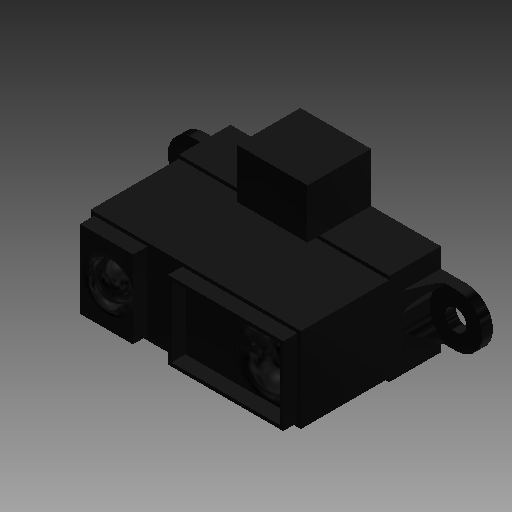
# Autodesk Inventor part: PSD
Saved by Autodesk Inventor 2017 (Build 210142000, 142)
## iProperties
Created: 2011-08-11
Part Number: PSD
Document SubType Name: Modeling
Designer: user
Density: 1.0545 g/cm^3
Mass: 5 g
Surface Area: 26.4147 cm^2
Volume: 4.74158 cm^3
Material: 알루미늄-6061
Appearance: 광택 - 검은색
Author: user
Autodesk Inventor part; units mm, degrees
ref_plane "YZ Plane" through (0, 0, 0) normal (1, 0, 0) x (0, 1, 0)
ref_plane "XZ Plane" through (0, 0, 0) normal (0, 1, 0) x (-1, 0, 0)
ref_plane "XY Plane" through (0, 0, 0) normal (0, 0, 1) x (1, 0, 0)
sketch "스케치1" plane through (0, 0, 0) normal (0, 0, 1) x (1, 0, 0)
  line L0 (0, 0) -> (-29.75, 0)
  line L1 (-29.75, 13) -> (0, 13)
  arc A0 (3.625, 2.75) -> (3.625, 10.25) centre (3.625, 6.5) ccw
  circle A1 centre (-33.375, 6.5) radius 1.5
  circle A2 centre (3.625, 6.5) radius 1.5
  line L2 (-0.25, 6.5) -> (0, 6.5)
  line L3 (-0.25, 6.5) -> (0, 6.5)
  line L4 (-37.125, 6.5) -> (-34.875, 6.5)
  line L5 (-29.5, 6.5) -> (-29.25, 6.5)
  line L6 (-29.75, 0) -> (-29.75, 2.75)
  line L7 (-29.75, 10.25) -> (-29.75, 13)
  arc A3 (-33.375, 10.25) -> (-33.375, 2.75) centre (-33.375, 6.5) ccw
  line L8 (-33.375, 10.25) -> (-29.75, 10.25)
  line L9 (0, 10.25) -> (3.625, 10.25)
  line L10 (3.625, 2.75) -> (0, 2.75)
  line L11 (-29.75, 2.75) -> (-33.375, 2.75)
  line L12 (0, 13) -> (0, 10.25)
  line L13 (0, 2.75) -> (0, 0)
  line L14 (5.125, 6.5) -> (7.375, 6.5)
  point P0 (-14.75, 6.5)
  point P1 (-14.75, 6.5)
  dimension "d5" = 3
  dimension "d56" = 3
  dimension "d0" = 29.75
  dimension "d1" = 13
  dimension "d3" = 7.5
  dimension "d4" = 44.5
  dimension "d53" = 29.75
  dimension "d54" = 2.125
  dimension "d55" = 2.125
  constraints: 30 end point, 9 parallel, 6 perpendicular, 6 point on circle, 3 horizontal, 2 centre point, 2 coincident, 2 horizontal alignment, 4 other
  measures "d0" distance of L1.start L1.end
  measures "d1" distance of L1.end L0.start
  measures "d3" diameter of A0
  measures "d4" distance of L4.start L14.end
  measures "d53" distance between parallel lines of L13 L6
extrude "돌출1" add sketch "스케치1" along normal blind 7.3
sketch "스케치2" plane through (0, 0, 7.3) normal (0, 0, 1) x (1, 0, 0)
  circle A0 centre (3.625, 6.5) radius 1.5 projected
  circle A1 centre (-33.375, 6.5) radius 1.5 projected
  line L0 (-29.75, 10.25) -> (-37, 10.25)
  line L1 (-37, 10.25) -> (-37, 0.8683)
  line L2 (-37, 0.8683) -> (-29.75, 0.8683)
  line L3 (-29.75, 0.8683) -> (-29.75, 10.25)
  line L4 (0, 10.25) -> (7.9641, 10.25)
  line L5 (7.9641, 10.25) -> (7.9641, 2.75)
  line L6 (7.9641, 2.75) -> (0, 2.75)
  line L7 (0, 2.75) -> (0, 10.25)
  constraints: 16 end point, 4 parallel, 2 horizontal, 2 perpendicular
extrude "돌출2" cut sketch "스케치2" against normal blind 5.8
chamfer "모따기1" distance 2 angle 45 2 edges at (0, 6.5, 1.5) (-29.75, 6.5, 1.5)
chamfer "모따기2" distance 2 angle 45 2 edges at (-29.75, 6.5, 3.5) (0, 6.5, 3.5)
sketch "스케치3" plane through (0, 0, 7.3) normal (0, 0, 1) x (1, 0, 0)
  line L0 (0, 13) -> (0, 0) projected
  line L1 (-29.75, 0) -> (-29.75, 13) projected
  line L2 (-29.75, 6.5) -> (0, 6.5)
  line L3 (0, 6.5) -> (0, 12.5)
  line L4 (0, 12.5) -> (-29.75, 12.5)
  line L5 (-29.75, 12.5) -> (-29.75, 6.5)
  line L6 (0, 12.5) -> (-29.75, 12.5)
  line L7 (-29.75, 12.5) -> (-29.75, 0.5)
  line L8 (-29.75, 0.5) -> (0, 0.5)
  line L9 (0, 0.5) -> (0, 12.5)
  dimension "d17" = 6
  dimension "d57" = 6
  constraints: 16 end point, 4 parallel, 2 horizontal, 2 perpendicular, 2 point on line, 1 midpoint
  measures "d17" distance of L4.end L2.start
  measures "d57" distance between parallel lines of L8 L2
extrude "돌출3" add sketch "스케치3" along normal blind 14.5
sketch "스케치4" plane through (0, 0, 21.8) normal (0, 0, 1) x (1, 0, 0)
  line L0 (-29.75, 0.5) -> (-29.75, 12.5) projected
  line L1 (0, 0.5) -> (-29.75, 0.5) projected
  line L2 (0, 12.5) -> (0, 0.5) projected
  line L3 (-29.75, 12.5) -> (0, 12.5) projected
  line L4 (-29.25, 12) -> (-0.5, 12)
  line L5 (-0.5, 12) -> (-0.5, 1)
  line L6 (-0.5, 1) -> (-29.25, 1)
  line L7 (-29.25, 1) -> (-29.25, 12)
  line L8 (-29.25, 12) -> (-21.75, 12)
  line L9 (-21.75, 12) -> (-21.75, 1)
  line L10 (-21.75, 1) -> (-29.25, 1)
  line L11 (-29.25, 1) -> (-29.25, 12)
  line L12 (-0.5, 12) -> (-16.8, 12)
  line L13 (-16.8, 12) -> (-16.8, 1)
  line L14 (-16.8, 1) -> (-0.5, 1)
  line L15 (-0.5, 1) -> (-0.5, 12)
  point P0 (0, 0)
  dimension "d22" = 0.5
  dimension "d23" = 0.5
  dimension "d24" = 0.5
  dimension "d25" = 0.5
  dimension "d26" = 7.5
  dimension "d27" = 16.3
  constraints: 24 end point, 6 parallel, 3 horizontal, 3 perpendicular, 2 point on line
  measures "d22" distance between parallel lines of L2 L5
  measures "d23" distance between parallel lines of L0 L7
  measures "d24" distance between parallel lines of L6 L1
  measures "d25" distance between parallel lines of L3 L4
  measures "d26" distance of L4.start L8.end
  measures "d27" distance of L4.end L12.end
extrude "돌출4" cut sketch "스케치4" against normal blind 2 contours L0 L3 L2 L1 | L4 L13 L6 L9
sketch "스케치5" plane through (0, 0, 21.8) normal (0, 0, 1) x (1, 0, 0)
  line L0 (-0.5, 1) -> (-0.5, 12) projected
  line L1 (-0.5, 12) -> (-16.8, 12) projected
  line L2 (-16.8, 12) -> (-16.8, 1) projected
  line L3 (-16.8, 1) -> (-0.5, 1) projected
  line L4 (-16.3, 11.5) -> (-1, 11.5)
  line L5 (-1, 11.5) -> (-1, 1.5)
  line L6 (-1, 1.5) -> (-16.3, 1.5)
  line L7 (-16.3, 1.5) -> (-16.3, 11.5)
  line L8 (-29.25, 1) -> (-21.75, 1) projected
  line L9 (-21.75, 1) -> (-21.75, 12) projected
  line L10 (-21.75, 12) -> (-29.25, 12) projected
  line L11 (-29.25, 12) -> (-29.25, 1) projected
  circle A0 centre (-25.25, 6.5) radius 2.75
  point P0 (0, 0)
  dimension "d30" = 0.5
  dimension "d31" = 0.5
  dimension "d32" = 0.5
  dimension "d33" = 0.5
  dimension "d34" = 5.5
  constraints: 8 end point, 2 parallel, 1 centre point, 1 horizontal, 1 perpendicular
  measures "d30" distance between parallel lines of L0 L5
  measures "d31" distance between parallel lines of L1 L4
  measures "d32" distance between parallel lines of L7 L2
  measures "d33" distance between parallel lines of L6 L3
  measures "d34" diameter of A0
extrude "돌출5" cut sketch "스케치5" against normal blind 2 contours L4 L5 L6 L7 | A0
fillet "모깎기1" radius 1 1 edges at (-28, 6.5, 21.8)
sketch "스케치6" plane through (0, 0, 19.8) normal (0, 0, 1) x (1, 0, 0)
  line L0 (-1, 1.5) -> (-1, 11.5) projected
  circle A0 centre (-4.2, 6.5) radius 2.75
  point P0 (0, 0)
  dimension "d38" = 5.5
  dimension "d39" = 3.2
  constraints: 1 centre point
  measures "d38" diameter of A0
  measures "d39" distance from line of L0 A0.centre
extrude "돌출6" cut sketch "스케치6" against normal blind 4
fillet "모깎기2" radius 3 1 edges at (-6.95, 6.5, 19.8)
sketch "스케치7" plane through (-4.2, 6.5, 15.8) normal (0, 0, 1) x (1, 0, 0)
  circle A0 centre (0, 0) radius 2.75 projected
  line L0 (-2.75, 0) -> (2.75, 0)
  point P0 (4.2, -6.5)
  constraints: 2 end point, 2 point on circle, 1 horizontal
revolve "회전1" add sketch "스케치7" angle 360 about axis through (-6.95, 6.5, 15.8) along (1, 0, 0) picked at (-1.0422, 1.0339) contours L0 A0
sketch "스케치8" plane through (-25.25, 6.5, 19.8) normal (0, 0, 1) x (1, 0, 0)
  circle A0 centre (0, 0) radius 2.75 projected
  line L0 (0, -2.75) -> (0, 2.75)
  point P0 (25.25, -6.5)
  constraints: 2 end point, 2 point on circle, 1 vertical
revolve "회전2" add sketch "스케치8" angle 360 about axis through (-25.25, 3.75, 19.8) along (0, 1, 0) picked at (0.3977, 0.8259) contours A0 L0
sketch "스케치9" plane through (-29.75, 13, 0) normal (0, 1, 0) x (1, 0, 0)
  line L0 (29.75, 0) -> (0, 0) projected
  line L1 (14.875, 0) -> (19.875, 0)
  line L2 (19.875, 0) -> (19.875, -9)
  line L3 (19.875, -9) -> (14.875, -9)
  line L4 (14.875, -9) -> (14.875, 0)
  line L5 (19.875, -9) -> (9.875, -9)
  line L6 (9.875, -9) -> (9.875, 0)
  line L7 (9.875, 0) -> (19.875, 0)
  line L8 (19.875, 0) -> (19.875, -9)
  dimension "d45" = 10
  dimension "d46" = 5
  dimension "d47" = 9
  constraints: 16 end point, 4 parallel, 2 horizontal, 2 perpendicular, 1 midpoint, 1 point on line
  measures "d45" distance of L2.end L5.end
  measures "d46" distance of L2.end L3.end
  measures "d47" distance of L1.end L2.end
extrude "돌출7" add sketch "스케치9" along normal blind 7
sketch "스케치10" plane through (0, 0, 1.5) normal (0, 0, 1) x (1, 0, 0)
  circle A0 centre (-33.375, 6.5) radius 1.5 projected
  line L0 (2, 2.75) -> (2, 10.25) projected
  line L1 (3.625, 2.75) -> (2, 2.75) projected
  arc A1 (3.625, 2.75) -> (3.625, 10.25) centre (3.625, 6.5) ccw projected
  line L2 (2, 10.25) -> (3.625, 10.25) projected
  circle A2 centre (3.625, 6.5) radius 1.5 projected
  circle A3 centre (-33.375, 6.5) radius 3.75
  circle A4 centre (3.625, 6.5) radius 3.75
  line L3 (-0.5, 1) -> (-0.5, 12) projected
  line L4 (-16.8, 1) -> (-0.5, 1) projected
  line L5 (-16.8, 12) -> (-16.8, 1) projected
  line L6 (-0.5, 12) -> (-16.8, 12) projected
  line L7 (-29.25, 1) -> (-21.75, 1) projected
  line L8 (-29.25, 12) -> (-29.25, 1) projected
  line L9 (-21.75, 12) -> (-29.25, 12) projected
  line L10 (-21.75, 1) -> (-21.75, 12) projected
  line L11 (0, 0.5) -> (-29.75, 0.5) projected
  line L12 (0, 12.5) -> (0, 0.5) projected
  line L13 (-29.75, 0.5) -> (-29.75, 12.5) projected
  line L14 (0, 7.4601) -> (0, 5.5399)
  line L15 (-29.75, 7.4601) -> (-29.75, 5.5399)
  line L16 (-29.75, 12.5) -> (0, 12.5) projected
  point P0 (0, 0)
  dimension "d50" = 7.5
  constraints: 5 point on circle, 4 end point, 4 point on line, 2 centre point, 2 coincident
  measures "d50" diameter of A3
extrude "돌출8" cut sketch "스케치10" along normal blind 6.2 contours A4 L12 L0 | L0 A4 A1 | A3 L13 picked at (-30.4583, 6.5)
